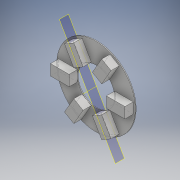
# Autodesk Inventor part: rotor-type2
Saved by Autodesk Inventor 2018 (Build 220112000, 112)
## iProperties
Created: 2025-02-23
Part Number: rotor-type2
Material: Generic
Document SubType Name: Modeling
Designer: neo
Density: 1 g/cm^3
Appearance: Default
Author: neo
Autodesk Inventor part; units mm, degrees
ref_plane "YZ Plane" through (0, 0, 0) normal (1, 0, 0) x (0, 1, 0)
ref_plane "XZ Plane" through (0, 0, 0) normal (0, 1, 0) x (-1, 0, 0)
ref_plane "XY Plane" through (0, 0, 0) normal (0, 0, 1) x (1, 0, 0)
sketch "Sketch1" plane through (0, 0, 0) normal (0, 1, 0) x (-1, 0, 0)
  line L0 (-2.439, 103.9756) -> (-2.439, -118.4634)
  line L1 (89.878, -0.9024) -> (-81.0976, -0.9024)
  line L2 (87.561, 12.0976) -> (42.561, 12.0976)
  line L3 (42.561, 12.0976) -> (42.561, -13.9024)
  line L4 (42.561, -13.9024) -> (87.561, -13.9024)
  line L5 (87.561, -13.9024) -> (87.561, 12.0976)
  line L6 (31.3026, 83.5398) -> (8.8026, 44.5687)
  line L7 (8.8026, 44.5687) -> (31.3193, 31.5687)
  line L8 (31.3193, 31.5687) -> (53.8193, 70.5398)
  line L9 (53.8193, 70.5398) -> (31.3026, 83.5398)
  line L10 (-58.6974, 70.5398) -> (-36.1974, 31.5687)
  line L11 (-36.1974, 31.5687) -> (-13.6807, 44.5687)
  line L12 (-13.6807, 44.5687) -> (-36.1807, 83.5398)
  line L13 (-36.1807, 83.5398) -> (-58.6974, 70.5398)
  line L14 (-92.439, -13.9024) -> (-47.439, -13.9024)
  line L15 (-47.439, -13.9024) -> (-47.439, 12.0976)
  line L16 (-47.439, 12.0976) -> (-92.439, 12.0976)
  line L17 (-92.439, 12.0976) -> (-92.439, -13.9024)
  line L18 (-36.1807, -85.3447) -> (-13.6807, -46.3736)
  line L19 (-13.6807, -46.3736) -> (-36.1974, -33.3736)
  line L20 (-36.1974, -33.3736) -> (-58.6974, -72.3447)
  line L21 (-58.6974, -72.3447) -> (-36.1807, -85.3447)
  line L22 (53.8193, -72.3447) -> (31.3193, -33.3736)
  line L23 (31.3193, -33.3736) -> (8.8026, -46.3736)
  line L24 (8.8026, -46.3736) -> (31.3026, -85.3447)
  line L25 (31.3026, -85.3447) -> (53.8193, -72.3447)
  point P0 (0, 0)
  point P1 (-2.439, -0.9024)
  point P2 (43.7195, 79.0465)
  point P3 (-48.5976, 79.0465)
  point P4 (-94.7561, -0.9024)
  point P5 (-48.5976, -80.8514)
  point P6 (43.7195, -80.8514)
  dimension "d0" = 180
  dimension "d1" = 26
  dimension "d3" = 90
  dimension "d6" = 360
  constraints: 52 end point, 2 horizontal, 2 parallel, 2 point on line, 1 perpendicular, 1 vertical, 56 other
  measures "d0" diameter of L5 L0
  measures "d1" distance between parallel lines of L2 L4
  measures "d3" diameter of L3 L0
extrude "Extrusion1" add sketch "Sketch1" along normal blind 20
sketch "Sketch2" plane through (-8.8026, 0, -46.3736) normal (0.5, 0, 0.866) x (0.866, 0, -0.5)
  line L0 (-26, 0) -> (0, 0) projected
  line L1 (0, 0) -> (0, 20) projected
  line L2 (-26, 20) -> (0, 20) projected
  line L3 (-26, 0) -> (-26, 20) projected
  line L4 (-23, 23) -> (0, 0)
  line L5 (-26, 20) -> (0, 20) projected
  line L6 (-23, -3) -> (0, 20)
  point P0 (-15.5635, 0)
  point P1 (-11.6957, 8.3043)
  constraints: 2 end point, 5 other
extrude "Extrusion2" [suppressed]
pattern_circular "Circular Pattern1" [suppressed]
ref_plane "Work Plane1" through (24.939, 0, -39.8736) normal (-0.866, 0, -0.5) x (-0.5, 0, 0.866)
sketch "Sketch3" plane through (24.939, 0, -39.8736) normal (-0.866, 0, -0.5) x (-0.5, 0, 0.866)
  line L0 (45, 26.4) -> (45, -4.4) projected
  line L1 (0, 20) -> (-50, 20)
  line L2 (-50, 20) -> (-50, 22)
  line L3 (-50, 22) -> (0, 22)
  line L4 (0, 22) -> (0, 20)
  line L5 (-11.2583, 20) -> (11.2583, 20) projected
  point P0 (47.001, 0)
  dimension "d16" = 90
  dimension "d18" = 2
  dimension "d19" = 0
  dimension "d21" = 190
  constraints: 8 end point, 2 parallel, 1 horizontal, 1 perpendicular
  measures "d16" diameter of L4 L0
  measures "d18" distance of L3.end L1.start
  measures "d19" distance between parallel lines of L5 L1
  measures "d21" diameter of L2 L0
revolve "Revolution1" add sketch "Sketch3" angle 360 about axis through (2.439, 0, -0.9024) along (0, -1, 0)
body "Solid1"
